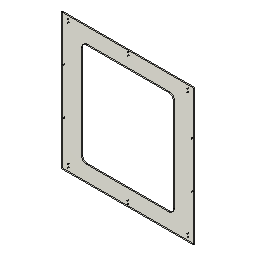
enclosure-front250 v23 (Autodesk Fusion 360 design; units mm, degrees)
Autodesk Fusion 360 part; units mm, degrees
sketch "Sketch1" plane through (0, 0, 0) normal (0, 0, 1) x (1, 0, 0)
  line L0 (284.2, -291.299) -> (-284.2, -291.299)
  line L1 (-284.2, -291.299) -> (-284.2, 291.299)
  line L2 (-284.2, 291.299) -> (284.2, 291.299)
  line L3 (284.2, 291.299) -> (284.2, -291.299)
  line L4 (284.2, -291.299) -> (-284.2, 291.299) construction
  line L5 (-284.2, -291.299) -> (284.2, 291.299) construction
  line L6 (-261.35, 291.299) -> (-261.35, -291.299) construction
  circle A0 centre (-261.35, 280.639) radius 2
  circle A1 centre (-261.35, 266.5) radius 2
  circle A2 centre (-261.35, -280.639) radius 2
  circle A3 centre (-261.35, -266.5) radius 2
  line L7 (261.35, 291.299) -> (261.35, -291.299) construction
  circle A4 centre (261.35, 280.639) radius 2
  circle A5 centre (261.35, 266.5) radius 2
  circle A6 centre (261.35, -280.639) radius 2
  circle A7 centre (261.35, -266.5) radius 2
  line L8 (-261.35, -266.5) -> (261.35, -266.5) construction
  circle A8 centre (0, -273.16) radius 2
  line L9 (0, -291.299) -> (0, 291.299) construction
  circle A9 centre (0, 273.16) radius 2
  circle A10 centre (0, 287.299) radius 2
  circle A11 centre (0, -287.299) radius 2
  line L10 (200, 225) -> (-200, 225)
  line L11 (-200, 225) -> (-200, -225)
  line L12 (-200, -225) -> (200, -225)
  line L13 (200, -225) -> (200, 225)
  line L14 (200, 225) -> (-200, -225) construction
  line L15 (-200, 225) -> (200, -225) construction
  line L16 (-289.2, 296.299) -> (289.2, 296.299)
  line L17 (289.2, 296.299) -> (289.2, -296.299)
  line L18 (289.2, -296.299) -> (-289.2, -296.299)
  line L19 (-289.2, -296.299) -> (-289.2, 296.299)
  circle A12 centre (279.2, 101.299) radius 2
  circle A13 centre (279.2, -101.299) radius 2
  circle A14 centre (-279.2, -101.299) radius 2
  circle A15 centre (-279.2, 101.299) radius 2
  line L20 (-304.8, -372.499) -> (304.8, -372.499) construction
  line L21 (304.8, -372.499) -> (304.8, 541.901) construction
  line L22 (304.8, 541.901) -> (-304.8, 541.901) construction
  line L23 (-304.8, 541.901) -> (-304.8, -372.499) construction
  line L24 (0, -372.499) -> (0, -296.299) construction
  line L25 (-261.35, 266.5) -> (261.35, 266.5) construction
  line L26 (261.35, -280.639) -> (-261.35, -280.639) construction
  line L27 (261.35, 280.639) -> (-261.35, 280.639) construction
  dimension "d1" = 568.4
  dimension "d2" = 582.598
  dimension "d3" = 22.85
  dimension "d4" = 4
  dimension "d6" = 4
  dimension "d8" = 4
  dimension "d9" = 4
  dimension "d12" = 22.85
  dimension "d13" = 4
  dimension "d14" = 4
  dimension "d17" = 4
  dimension "d18" = 4
  dimension "d21" = 4
  dimension "d22" = 4
  dimension "d23" = 4
  dimension "d24" = 4
  dimension "d28" = 450
  dimension "d29" = 400
  dimension "d30" = 5
  dimension "d31" = 5
  dimension "d32" = 5
  dimension "d33" = 5
  dimension "d37" = 4
  dimension "d38" = 4
  dimension "d39" = 4
  dimension "d40" = 4
  dimension "d41" = 190
  dimension "d42" = 190
  dimension "d43" = 5
  dimension "d44" = 5
  dimension "d45" = 190
  dimension "d46" = 190
  dimension "d47" = 5
  dimension "d49" = 5
  dimension "d51" = 609.6
  dimension "d52" = 76.2
  dimension "d53" = 914.4
  dimension "d54" = 24.799
  dimension "d55" = 24.799
  dimension "d56" = 10.66
  dimension "d57" = 10.66
  dimension "d61" = 4
  dimension "d62" = 14.139
  dimension "d63" = 14.139
  dimension "d64" = 4
  measures "d3" distance of L1 L6
  measures "d4" diameter of A0
  measures "d6" diameter of A1
  measures "d8" diameter of A2
  measures "d9" diameter of A3
  measures "d12" distance of L3 L7
  measures "d13" diameter of A4
  measures "d14" diameter of A5
  measures "d17" diameter of A6
  measures "d18" diameter of A7
  measures "d21" diameter of A8
  measures "d22" diameter of A9
  measures "d23" diameter of A10
  measures "d24" diameter of A11
  measures "d30" distance of L3 L17
  measures "d31" distance of L1 L19
  measures "d32" distance of L2 L16
  measures "d33" distance of L0 L18
  measures "d37" diameter of A12
  measures "d38" diameter of A13
  measures "d39" diameter of A14
  measures "d40" diameter of A15
  measures "d54" distance of L2 L25
  measures "d55" distance of L0 L8
  measures "d56" distance of L0 L26
  measures "d57" distance of L2 L27
extrude "Extrude1" add sketch "Sketch1" along normal blind 5 contours L0 L1 L2 L3 | L16 L17 L18 L19 makes body 1
fillet "Fillet1" radius 20 4 edges at (-200, -225, 2.5) (200, -225, 2.5) (200, 225, 2.5) (-200, 225, 2.5) on bodies 1
copy_body "Body->Comp1" bodies 1 removing the originals makes body 2 in component "Front Panel"
component "Front Panel" placed x (1, 0, 0) y (0, 1, 0) z (0, 0, 1) at (0, 0, 0)
equation "d1 = XRailLength + 218.4 mm"
equation "d2 = PrintHeight + 282.598 mm"
equation "d28 = PrintHeight + 150 mm"
equation "d29 = XRailLength + 50 mm"
equation "d30 = WallThickness"
equation "d31 = WallThickness"
equation "d32 = WallThickness"
equation "d33 = WallThickness"
equation "WallThickness = 5 mm"
equation "XRailLength = 350 mm"
equation "PrintHeight = 300 mm"
named bodies: "Front Panel"
